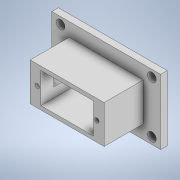
# Autodesk Inventor part: ServoESP32_V3Base
Saved by Autodesk Inventor 2020 (Build 240168000, 168)
## iProperties
Created: 2022-11-23
Part Number: ServoESP32_V3Base
Material: Generic
Document SubType Name: Modeling
Designer: chava4445
Density: 1 g/cm^3
Appearance: Default
Author: chava4445
## iProperties of the stored document _3DPrint.ipt
Created: 2022-12-01
Part Number: _3DPrint
Material: Generic
Document SubType Name: Modeling
Designer: agraa4529
Density: 1 g/cm^3
Appearance: Default
Author: agraa4529
Autodesk Inventor part; units mm, degrees
ref_plane "YZ Plane" through (0, 0, 0) normal (1, 0, 0) x (0, 1, 0)
ref_plane "XZ Plane" through (0, 0, 0) normal (0, 1, 0) x (-1, 0, 0)
ref_plane "XY Plane" through (0, 0, 0) normal (0, 0, 1) x (1, 0, 0)
sketch "Sketch1" plane through (0, 0, 0) normal (0, 0, 1) x (1, 0, 0)
  point P0 (0, 0)
sketch "Sketch2" plane through (0, 0, 0) normal (0, 0, 1) x (1, 0, 0)
  line L0 (-25, 15) -> (25, 15)
  line L1 (25, 15) -> (25, -15)
  line L2 (25, -15) -> (-25, -15)
  line L3 (-25, -15) -> (-25, 15)
  line L4 (-25, 15) -> (25, -15) construction
  line L5 (25, 15) -> (-25, -15) construction
  point P0 (0, 0)
  dimension "d0" = 30
  dimension "d1" = 50
  constraints: 12 end point, 2 midpoint, 2 parallel, 1 horizontal, 1 perpendicular
  measures "d0" distance of L0.end L1.end
  measures "d1" distance of L0.start L0.end
extrude "Extrusion1" add sketch "Sketch2" along normal blind 3
sketch "Sketch3" plane through (0, 0, 3) normal (0, 0, 1) x (1, 0, 0)
  line L0 (-7.2947, 3.9789) -> (7.2947, -3.9789) construction
  line L1 (7.2947, 3.9789) -> (-7.2947, -3.9789) construction
  line L2 (-12.1, 7) -> (12.1, 7)
  line L3 (12.1, 7) -> (12.1, -7)
  line L4 (12.1, -7) -> (-12.1, -7)
  line L5 (-12.1, -7) -> (-12.1, 7)
  line L6 (-12.1, 7) -> (12.1, -7) construction
  line L7 (12.1, 7) -> (-12.1, -7) construction
  line L8 (-17, 8.75) -> (17, 8.75)
  line L9 (17, 8.75) -> (17, -8.75)
  line L10 (17, -8.75) -> (-17, -8.75)
  line L11 (-17, -8.75) -> (-17, 8.75)
  line L12 (-17, 8.75) -> (17, -8.75) construction
  line L13 (17, 8.75) -> (-17, -8.75) construction
  point P0 (0, 0)
  dimension "d4" = 24.2
  dimension "d5" = 14
  dimension "d6" = 34
  dimension "d7" = 17.5
  constraints: 28 end point, 6 midpoint, 4 parallel, 2 horizontal, 2 perpendicular
  measures "d4" distance of L2.start L2.end
  measures "d5" distance of L2.end L3.end
  measures "d6" distance of L8.start L8.end
  measures "d7" distance of L8.end L9.end
extrude "Extrusion2" add sketch "Sketch3" along normal blind 18
sketch "Sketch5" plane through (-17, -8.75, 3) normal (-1, 0, 0) x (0, 0, 1)
  line L0 (0, 15.75) -> (0, 1.75) projected
  line L1 (0, 8.75) -> (14, 8.75) construction
  line L2 (2, 11.25) -> (12, 11.25)
  line L3 (12, 11.25) -> (12, 6.25)
  line L4 (12, 6.25) -> (2, 6.25)
  line L5 (2, 6.25) -> (2, 11.25)
  line L6 (2, 11.25) -> (12, 6.25) construction
  line L7 (12, 11.25) -> (2, 6.25) construction
  point P0 (-3, 8.75)
  point P1 (7, 8.75)
  dimension "d10" = 14
  dimension "d11" = 5
  dimension "d12" = 10
  constraints: 14 end point, 4 midpoint, 2 horizontal, 2 parallel, 1 perpendicular
  measures "d10" distance of L1.start L1.end
  measures "d11" distance of L2.end L3.end
  measures "d12" distance of L3.end L4.end
extrude "Extrusion3" cut sketch "Sketch5" against normal blind 18
sketch "Sketch6" plane through (0, 0, 21) normal (0, 0, 1) x (1, 0, 0)
  line L0 (12.1, 7) -> (12.1, -7) projected
  line L1 (12.1, 0) -> (13.7, 0) construction
  circle A0 centre (13.7, 0) radius 1
  line L2 (0, 0) -> (0, -10.1411) construction
  line L3 (-12.1, 0) -> (-13.7, 0) construction
  circle A1 centre (-13.7, 0) radius 1
  dimension "d15" = 1.6
  dimension "d16" = 2
  constraints: 6 end point, 3 symmetric about line, 2 centre point, 2 coincident, 1 horizontal, 1 midpoint, 1 vertical, 1 other
  measures "d15" distance of L1.start L1.end
  measures "d16" diameter of A0
extrude "Extrusion4" cut sketch "Sketch6" against normal blind 5
sketch "Sketch7" plane through (0, 0, 3) normal (0, 0, 1) x (1, 0, 0)
  point P0 (0, 0)
sketch "Sketch8" plane through (0, 0, 3) normal (0, 0, 1) x (1, 0, 0)
  line L0 (0, 0) -> (6.4971, 0) construction
  line L1 (0, 0) -> (0, -4.6086) construction
  line L2 (25, 15) -> (-25, 15) projected
  line L3 (17, 8.75) -> (-17, 8.75) projected
  line L4 (25, 15) -> (17, 8.75) construction
  circle A0 centre (21, 11.875) radius 2
  circle A1 centre (21, -11.875) radius 2
  circle A2 centre (-21, 11.875) radius 2
  circle A3 centre (-21, -11.875) radius 2
  dimension "d19" = 4
  constraints: 6 end point, 4 centre point, 3 symmetric about line, 1 horizontal, 1 midpoint, 1 vertical, 3 other
  measures "d19" diameter of A0
extrude "Extrusion5" cut sketch "Sketch8" against normal blind 3
sketch "Sketch9" plane through (0, 0, 0) normal (0, 0, -1) x (-1, 0, 0)
  point P0 (0, 0)
sketch "Sketch10" plane through (0, 0, 3) normal (0, 0, 1) x (1, 0, 0)
  line L0 (0, 0) -> (-12.1, 0) construction
  line L1 (-12.1, -2.5) -> (-12.1, 2.5) projected
  circle A0 centre (-6.05, 0) radius 3.5
  line L2 (0, 0) -> (0, -3.071) construction
  circle A1 centre (6.05, 0) radius 3.5
  dimension "d24" = 7
  constraints: 4 end point, 2 centre point, 2 midpoint, 1 symmetric about line, 1 vertical, 1 other
  measures "d24" diameter of A0
extrude "Extrusion6" cut sketch "Sketch10" against normal blind 10
body "Solid1"
